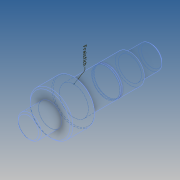
# Autodesk Inventor part: 200-40-BOGIE-CONNECTOR-05
Saved by Autodesk Inventor 2018.2 (Build 222227000, 227)
## iProperties
Manager: feesmrt
Company: FRANC0R
Created: 2017-12-05
Part Number: 200-40-BOGIE-CONNECTOR-05
Material: Aluminium 6061
Document SubType Name: Modeling
Designer: feesmrt
Density: 2.7 g/cm^3
Appearance: Aluminium - flach
Project: Rescue Robot
Cost Center: -
Engineer: feesmrt
Authority: feesmrt
Description: Bogie Connector Axle
Stock Number: 200-40-BOGIE-CONNECTOR-05
Author: feesmrt
Subject: Rescue Robot
Title: Bogie Connector Axle
Revision Number: 1
Autodesk Inventor part; units mm, degrees
ref_plane "YZ Plane" through (0, 0, 0) normal (1, 0, 0) x (0, 1, 0)
ref_plane "XZ Plane" through (0, 0, 0) normal (0, 1, 0) x (-1, 0, 0)
ref_plane "XY Plane" through (0, 0, 0) normal (0, 0, 1) x (1, 0, 0)
sketch "Skizze1" plane through (0, 0, 0) normal (1, 0, 0) x (0, 1, 0)
  line L0 (0, 17.7) -> (0, -2.95) construction
  line L1 (-59.5, 0) -> (59.5, 0) projected
  line L2 (42.5, 8) -> (42.5, 0)
  line L3 (42.5, 8) -> (27.5, 8)
  line L4 (27.5, 8) -> (27.5, 10)
  line L5 (27.5, 10) -> (-11.1, 10)
  line L6 (-11.1, 10) -> (-11.1, 14.75)
  line L7 (-11.1, 14.75) -> (-27.5, 14.75)
  line L8 (-27.5, 14.75) -> (-27.5, 8)
  line L9 (-27.5, 8) -> (-42.5, 8)
  line L10 (-42.5, 8) -> (-42.5, 0)
  line L11 (-11.1, 14.75) -> (11.1, 14.75) construction
  line L12 (11.1, 14.75) -> (11.1, 10) construction
  line L13 (-42.5, 0) -> (42.5, 0)
  point P0 (0, 0)
  dimension "d0" = 16
  dimension "d1" = 15
  dimension "d2" = 22.2
  dimension "d3" = 55
  dimension "d4" = 20
  dimension "d5" = 29.5
  constraints: 24 end point, 9 perpendicular, 3 point on line, 2 equal length, 2 horizontal, 1 collinear, 2 other
  measures "d0" diameter of L3 L1
  measures "d1" distance of L2.start L3.end
  measures "d2" distance between parallel lines of L12 L6
  measures "d3" distance between parallel lines of L4 L8
  measures "d4" diameter of L5 L1
  measures "d5" diameter of L7 L1
revolve "Grundkörper" add sketch "Skizze1" angle 360 about axis through (0, 0, 0) along (0, 1, 0)
sketch "Skizze2" plane through (0, 0, 0) normal (1, 0, 0) x (0, 1, 0)
  line L0 (-9.1, 0) -> (33.6, 0) construction
  line L1 (-11.1, -14.75) -> (-11.1, 14.75) construction
  line L2 (-11.1, 10) -> (27.5, 10) projected
  line L3 (-11.1, 10) -> (-11.1, 14.75)
  line L4 (-11.1, 14.75) -> (11.1, 14.75)
  line L5 (11.1, 14.75) -> (11.1, 10)
  line L6 (11.1, 10) -> (-11.1, 10)
  line L7 (0, 20.65) -> (0, -20.65) construction
  line L8 (11.1, 10) -> (11.1, 9.5)
  line L9 (11.1, 9.5) -> (12.4, 9.5)
  line L10 (12.4, 9.5) -> (12.4, 10)
  line L11 (11.1, 10) -> (12.4, 10)
  point P0 (0, 0)
  dimension "d15" = 1.3
  dimension "d16" = 19
  constraints: 16 end point, 4 perpendicular, 3 point on line, 2 collinear, 1 horizontal, 1 vertical, 1 other
  measures "d15" distance between parallel lines of L10 L8
  measures "d16" diameter of L9 L0
revolve "Nut_Sicherungsring_DIN471-20x1,2" cut sketch "Skizze2" angle 360 about axis through (0, 0, 0) along (0, 1, 0) contours L2 L10 L9 L8
chamfer "FaseAllgemein" distance 1 angle 45 3 edges at (0, -42.5, -8) (0, 42.5, -8) (0, -27.5, -14.75)
chamfer "FaseLager" distance 0.5 angle 45 1 edges at (0, -11.1, -14.75)
